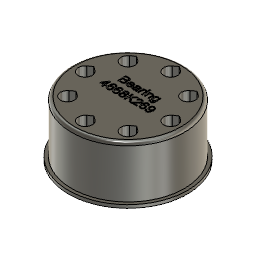
CarrierOutput (Autodesk Fusion 360 design; units mm, degrees)
Autodesk Fusion 360 part; units mm, degrees
sketch "Carrier" plane through (0, 0, 0) normal (0, 0, 1) x (1, 0, 0)
  circle A0 centre (0, 0) radius 17.375
  circle A1 centre (0, 0) radius 18.375
  dimension "d256" = 34.75
  dimension "d259" = 1
  constraint coincident A0.centre A1.centre
  measures "d256" diameter of A0
extrude "Extrude31" add sketch "Carrier" along normal blind 17 contours A0
extrude "Extrude32" add sketch "Carrier" along normal blind 1
fillet "Fillet12" radius 1 1 edges at (-16.1992, -6.2831, 17)
sketch "heat inserts" plane through (0, 0, 17) normal (0, 0, 1) x (-1, 0, 0)
  circle A0 centre (0, 0) radius 16.375
  line L0 (0, 0) -> (0, -13.2) construction
  circle A1 centre (0, -13.2) radius 2.15
  line L1 (-0.0013, -15.35) -> (-1.0012, -15.3494) construction
  line L2 (-0.0013, -15.35) -> (-0.0016, -15.85) construction
  line L3 (-0.0016, -15.85) -> (1.2559, -14.9451)
  line L4 (-0.0016, -15.85) -> (-1.2579, -14.9436)
  circle A2 centre (0, 0) radius 13.2 construction
  line L5 (9.9706, 4.912) -> (-9.824, 4.912) construction
  line L6 (-9.824, 4.912) -> (-9.824, -5.1319) construction
  line L7 (-9.824, -5.1319) -> (9.9706, -5.1319) construction
  line L8 (9.9706, -5.1319) -> (9.9706, 4.912) construction
  dimension "d264" = 13.2
  dimension "d265" = 4.3
  dimension "d283" = 0.5
  dimension "d284" = 26.4
  dimension "d349" = 2.5
  text T0 "Bearing 4668K269" font "Arial" height 2.5 align centre top in box 19.7946 x 10.0439 at (9.9706, 4.912) x (-1, 0) y (0, -1) spacing 1
  constraint vertical L0
  constraint coincident A0.centre L0.start
  constraint coincident L0.end A1.centre
  constraint coincident A1 L1.start
  constraint tangent A1 L1
  constraint perpendicular L1 L2
  constraint coincident A1 L3.end
  constraint tangent A1 L3
  constraint symmetric L3.start L2 L4.start
  constraint symmetric L2 L3.end L4.end
  measures "d264" distance of A0.centre L0.end
  measures "d265" diameter of A1
  measures "d283" distance of L1.start L2.end
  measures "d284" diameter of A2
extrude "Extrude33" cut sketch "heat inserts" against normal blind 12 contours A1 | A1 L3 L4
pattern_path "PathPattern1" count 8 spacing 10.3673 from (0, 13.2, 17) path "heat inserts" along A2 of "Extrude33"
extrude "Extrude35" cut sketch "heat inserts" against normal blind 1 text T0
equation "bearing_mount_lip = 1 mm"
equation "m3 = 3.05 mm"
equation "heat_insert_diameter = 4.3 mm"
equation "bolt_circle_radius = ( bearing_ID / 2 ) - heat_insert_diameter"
equation "n_heat_insert = 8"
equation "height = bearing_width + 10 mm"
equation "heat_insert_depth = 12 mm"
equation "d256 = bearing_ID + bearing_id_fit"
equation "d257 = height"
equation "d260 = bearing_mount_lip"
equation "d264 = bolt_circle_radius"
equation "d265 = heat_insert_diameter"
equation "d266 = -heat_insert_depth"
equation "bearing_id_fit = -0.25 mm"
equation "d284 = bolt_circle_diameter"
equation "d285 = n_heat_insert"
equation "d286 = bolt_circle_radius * 2 * PI / n_heat_insert"
equation "bolt_circle_diameter = bolt_circle_radius * 2"
equation "gear_ratio = 6"
equation "sun_teeth = if(is_Nema_17 == 1; 12; 15)"
equation "ring_teeth = ( gear_ratio - 1 ) * sun_teeth"
equation "gear_OD = ( ring_teeth * module * diameter_scale ) + ring_thickness"
equation "thickness = 2 mm"
equation "m3_pilot = 3.3 mm"
equation "bearing_OD = if(max_bearing_OD < 47 mm - 1E-06 mm; bearing_5972K282_OD; if(max_bearing_OD < 52 mm - 1E-06 mm; bearing_4668K269_OD; if(max_bearing_OD < 58 mm - 1E-06 mm; bearing_4668K271_OD; if(max_bearing_OD < 65 mm - 1E-06 mm; bearing_4668K272_OD; if(max_bearing_OD < 72 mm - 1E-06 mm; bearing_4668K273_OD; if(max_bearing_OD < 78 mm - 1E-06 mm; bearing_6656K146_OD; if(max_bearing_OD < 85 mm - 1E-06 mm; bearing_6656K148_OD; if(max_bearing_OD < 90 mm - 1E-06 mm; bearing_6656K238_OD; if(max_bearing_OD < 95 mm - 1E-06 mm; bearing_6656K241_OD; if(max_bearing_OD < 100 mm - 1E-06 mm; bearing_6656K243_OD; 0 mm))))))))))"
equation "wall_thickness = 6 mm"
equation "bearing_mount_clearance = 0.1 mm"
equation "bearing_width = ( if(( bearing_OD >= 42 mm ) and ( bearing_OD <= 65 mm ); 7; if(( bearing_OD >= 78 mm ) and ( bearing_OD <= 95 mm ); 10; 9)) ) * 1 mm"
equation "bearing_mount_wall_thickness = 2 mm"
equation "bearing_mount_lip_height = 2 mm"
equation "m3_inserts_diameter = 4.3 mm"
equation "m3_inserts_wall_thickness = 1.8 mm"
equation "m3_head_diameter = 5.2 mm + 0.2 mm"
equation "m3_head_height = 3 mm"
equation "m3_chamfer = 1 mm"
equation "module = 1"
equation "helix_angle = 0 deg"
equation "diameter_scale = ( 1 / cos(helix_angle) ) * 1 mm"
equation "is_Nema_17 = 1"
equation "ring_thickness = 8 mm"
equation "bearing_distance_from_edge = 21 mm"
equation "max_bearing_OD = gear_OD - bearing_distance_from_edge"
equation "bearing_5972K282_ID = 30 mm"
equation "bearing_5972K282_OD = 42 mm"
equation "bearing_5972K282_W = 7 mm"
equation "bearing_4668K269_ID = 35 mm"
equation "bearing_4668K269_OD = 47 mm"
equation "bearing_4668K269_W = 7 mm"
equation "bearing_4668K271_ID = 40 mm"
equation "bearing_4668K271_OD = 52 mm"
equation "bearing_4668K271_W = 7 mm"
equation "bearing_4668K272_ID = 45 mm"
equation "bearing_4668K272_OD = 58 mm"
equation "bearing_4668K272_W = 7 mm"
equation "bearing_4668K273_ID = 50 mm"
equation "bearing_4668K273_OD = 65 mm"
equation "bearing_4668K273_W = 7 mm"
equation "bearing_6656K146_ID = 55 mm"
equation "bearing_6656K146_OD = 72 mm"
equation "bearing_6656K146_W = 9 mm"
equation "bearing_6656K148_ID = 60 mm"
equation "bearing_6656K148_OD = 78 mm"
equation "bearing_6656K148_W = 10 mm"
equation "bearing_6656K241_ID = 70 mm"
equation "bearing_6656K241_OD = 90 mm"
equation "bearing_6656K241_W = 10 mm"
equation "bearing_6656K238_ID = 65 mm"
equation "bearing_6656K238_OD = 85 mm"
equation "bearing_6656K238_W = 10 mm"
equation "bearing_6656K243_ID = 75 mm"
equation "bearing_6656K243_OD = 95 mm"
equation "bearing_6656K243_W = 10 mm"
equation "bearing_ID = ( if(bearing_OD == 42 mm; 30; if(bearing_OD == 47 mm; 35; if(bearing_OD == 52 mm; 40; if(bearing_OD == 58 mm; 45; if(bearing_OD == 65 mm; 50; if(bearing_OD == 72 mm; 55; if(bearing_OD == 78 mm; 60; if(bearing_OD == 85 mm; 65; if(bearing_OD == 90 mm; 70; if(bearing_OD == 95 mm; 75; 0)))))))))) ) * 1 mm"
equation "bearing_part_number = if(max_bearing_OD < 47 mm - 1E-06 mm; '5972K282'; if(max_bearing_OD < 52 mm - 1E-06 mm; '4668K269'; if(max_bearing_OD < 58 mm - 1E-06 mm; '4668K271'; if(max_bearing_OD < 65 mm - 1E-06 mm; '4668K272'; if(max_bearing_OD < 72 mm - 1E-06 mm; '4668K273'; if(max_bearing_OD < 78 mm - 1E-06 mm; '6656K146'; if(max_bearing_OD < 85 mm - 1E-06 mm; '6656K148'; if(max_bearing_OD < 90 mm - 1E-06 mm; '6656K238'; if(max_bearing_OD < 95 mm - 1E-06 mm; '6656K241'; if(max_bearing_OD < 100 mm - 1E-06 mm; '6656K243'; '0 mm'))))))))))"
equation "d350 = 'Bearing ' + bearing_part_number"
